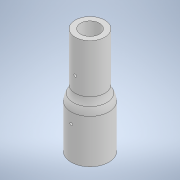
# Autodesk Inventor part: hollowCylinderTest
Saved by Autodesk Inventor 2022 (Build 260153000, 153)
## iProperties
Created: 2021-09-16
Part Number: hollowCylinderTest
Material: Generic
Document SubType Name: Modeling
Designer: tecware
Density: 1 g/cm^3
Appearance: Default
Author: tecware
## iProperties of the stored document hollowCylinderTest_3DPrint.ipt
Created: 2021-09-16
Part Number: hollowCylinderTest_3DPrint
Material: Generic
Document SubType Name: Modeling
Designer: tecware
Density: 1 g/cm^3
Appearance: Default
Author: tecware
Autodesk Inventor part; units mm, degrees
ref_plane "YZ Plane" through (0, 0, 0) normal (1, 0, 0) x (0, 1, 0)
ref_plane "XZ Plane" through (0, 0, 0) normal (0, 1, 0) x (-1, 0, 0)
ref_plane "XY Plane" through (0, 0, 0) normal (0, 0, 1) x (1, 0, 0)
sketch "Sketch1" plane through (0, 0, 0) normal (0, 1, 0) x (-1, 0, 0)
  circle A0 centre (0, 0) radius 7.15
  circle A1 centre (0, 0) radius 11.15
  point P0 (0, 11.15)
  dimension "d1" = 22.3
  dimension "d0" = 14.3
  constraints: 2 coincident, 1 centre point, 1 vertical alignment, 2 other
  measures "d0" diameter of A0
extrude "Small" add sketch "Sketch1" along normal blind 40
sketch "Sketch2" plane through (0, 0, 0) normal (0, -1, 0) x (1, 0, 0)
  circle A0 centre (0, 0) radius 7.15 projected
  circle A1 centre (0, 0) radius 10.2
  circle A2 centre (0, 0) radius 11.15 projected
  circle A3 centre (0, 0) radius 14.2
  point P0 (0, 14.2)
  dimension "d5" = 28.4
  dimension "d4" = 20.4
  constraints: 2 coincident, 1 centre point, 1 vertical alignment, 2 other
  measures "d4" diameter of A1
extrude "Big" add sketch "Sketch2" along normal blind 40 contours A2 | A3
ref_plane "Work Plane1" through (0, 0, 11.15) normal (0, 0, 1) x (1, 0, 0)
ref_plane "Work Plane2" through (0, 0, 14.2) normal (0, 0, 1) x (1, 0, 0)
sketch "Sketch3" plane through (0, 0, 11.15) normal (0, 0, 1) x (1, 0, 0)
  point P0 (0, 0)
  point P1 (0, 15)
hole "Screw Hole for small" at (0, 15, 11.15) direction (0, 0, -1) diameter 2 end through all
sketch "Sketch4" plane through (0, 0, 14.2) normal (0, 0, 1) x (1, 0, 0)
  point P0 (0, 0)
  point P1 (0, -15)
hole "Screw Hole for big" at (0, -15, 14.2) direction (0, 0, -1) diameter 2 end through all
fillet "Fillet1" radius 10 2 edges at (-14.2, 0, 0) (11.15, 0, 0)
body "Solid1"
